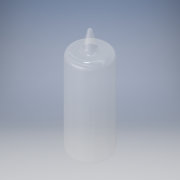
# Autodesk Inventor part: IN-14
Saved by Autodesk Inventor 2017 (Build 210142000, 142)
## iProperties
Created: 2017-04-18
Part Number: IN-14
Material: Generic
Document SubType Name: Modeling
Designer: jeffkub
Density: 1 g/cm^3
Appearance: Clear(1)
Author: jeffkub
Autodesk Inventor part; units mm, degrees
ref_plane "YZ Plane" through (0, 0, 0) normal (1, 0, 0) x (0, 1, 0)
ref_plane "XZ Plane" through (0, 0, 0) normal (0, 1, 0) x (-1, 0, 0)
ref_plane "XY Plane" through (0, 0, 0) normal (0, 0, 1) x (1, 0, 0)
sketch "Sketch1" plane through (0, 0, 0) normal (0, 0, 1) x (1, 0, 0)
  line L0 (0, 0) -> (-6.5, 0)
  line L1 (-9.5, 3) -> (-9.5, 42)
  arc A0 (0, 54.5) -> (-0.9781, 53.7079) centre (0, 53.5) ccw
  line L2 (-0.9781, 53.7079) -> (-2.4923, 46.5842)
  line L3 (-6.5, 45) -> (-4.4486, 45)
  arc A1 (-4.4486, 45) -> (-2.4923, 46.5842) centre (-4.4486, 47) ccw
  arc A2 (-6.5, 45) -> (-9.5, 42) centre (-6.5, 42) ccw
  arc A3 (-9.5, 3) -> (-6.5, 0) centre (-6.5, 3) ccw
  line L4 (0, 63.3885) -> (0, -6.2417)
  point P0 (0, 0)
  dimension "d0" = 2
  dimension "d1" = 3
  dimension "d2" = 45
  dimension "d3" = 1
  dimension "d5" = 53.5
  dimension "d7" = 12
  dimension "d8" = 19
  constraints: 10 end point, 8 point on circle, 7 tangent, 4 centre point, 3 point on line, 1 coincident, 1 equal radius, 1 horizontal, 1 parallel, 1 vertical, 1 vertical alignment
  measures "d0" radius of A1
  measures "d1" radius of A2
  measures "d2" distance between parallel lines of L0 L3
  measures "d3" radius of A0
  measures "d5" distance from line of L0 A0.centre
  measures "d7" angle of L4 L2
  measures "d8" diameter of L1 L4
revolve "Revolution1" add sketch "Sketch1" angle 360 about axis through (0, 63.3885, 0) along (0, -1, 0)
body "Solid1"
